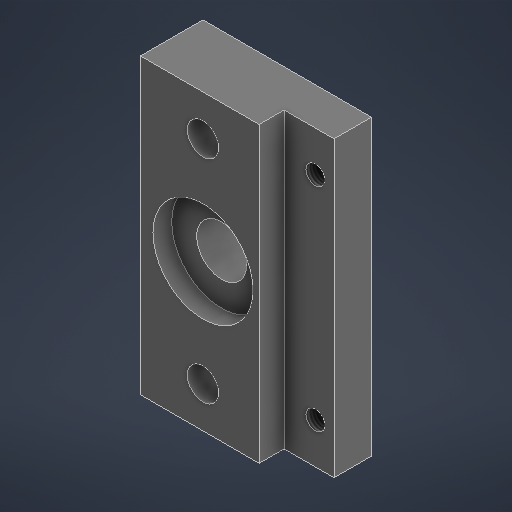
# Autodesk Inventor part: Szorítólap
Saved by Autodesk Inventor 2025 (Build 290162010, 162A)
## iProperties
Created: 2025-02-13
Part Number: Szorítólap
Material: Generic
Document SubType Name: Modeling
Designer: petruska.milan
Density: 1 g/cm^3
Appearance: Gray
Author: petruska.milan
Autodesk Inventor part; units mm, degrees
ref_plane "YZ Plane" through (0, 0, 0) normal (1, 0, 0) x (0, 1, 0)
ref_plane "XZ Plane" through (0, 0, 0) normal (0, 1, 0) x (-1, 0, 0)
ref_plane "XY Plane" through (0, 0, 0) normal (0, 0, 1) x (1, 0, 0)
sketch "Sketch1" plane through (0, 0, 0) normal (0, 0, 1) x (1, 0, 0)
  line L0 (-13.5, -23.5) -> (13.5, -23.5)
  line L1 (13.5, -23.5) -> (13.5, 23.5)
  line L2 (13.5, 23.5) -> (-13.5, 23.5)
  line L3 (-13.5, 23.5) -> (-13.5, -23.5)
  line L4 (-13.5, -23.5) -> (13.5, 23.5) construction
  line L5 (13.5, -23.5) -> (-13.5, 23.5) construction
  point P0 (0, 0)
  dimension "d0" = 27
  dimension "d1" = 47
  constraints: 12 end point, 2 midpoint, 2 parallel, 1 horizontal, 1 perpendicular
  measures "d0" distance of L2.end L1.end
  measures "d1" distance of L1.end L0.end
extrude "Extrusion1" add sketch "Sketch1" along normal blind 10
sketch "Sketch2" plane through (0, 0, 10) normal (0, 0, 1) x (1, 0, 0)
  line L0 (13.5, -23.5) -> (13.5, 23.5) projected
  line L1 (13.5, 23.5) -> (10.5, 23.5)
  line L2 (13.5, 23.5) -> (-13.5, 23.5) projected
  line L3 (10.5, 23.5) -> (10.5, 17)
  line L4 (10.5, 17) -> (10.5, -17)
  circle A0 centre (10.5, -17) radius 1.5
  circle A1 centre (10.5, 17) radius 1.5
  line L5 (13.5, 23.5) -> (10.5, 23.5)
  line L6 (13.5, 23.5) -> (-3.5, 23.5)
  line L7 (-3.5, 23.5) -> (-3.5, 17)
  circle A2 centre (-3.5, 17) radius 2.5
  line L8 (-3.5, 23.5) -> (-3.5, 0)
  circle A3 centre (-3.5, 0) radius 4
  line L9 (-3.5, 0) -> (-3.5, -15.5)
  line L10 (-3.5, -15.5) -> (-3.5, -17)
  circle A4 centre (-3.5, -17) radius 2.5
  point P0 (0, 0)
  dimension "d4" = 3
  dimension "d5" = 6.5
  dimension "d6" = 34
  dimension "d7" = 3
  dimension "d8" = 3
  dimension "d9" = 17
  dimension "d10" = 6.5
  dimension "d11" = 5
  dimension "d12" = 8
  dimension "d13" = 5
  constraints: 18 end point, 5 centre point, 5 coincident, 3 point on line, 3 vertical, 2 perpendicular, 1 collinear
  measures "d4" distance of L0.end L1.end
  measures "d5" distance of L1.end L3.end
  measures "d6" distance of L3.end L4.end
  measures "d7" diameter of A0
  measures "d8" diameter of A1
  measures "d9" distance of L0.end L6.end
  measures "d10" distance of L6.end L7.end
  measures "d11" diameter of A2
  measures "d12" diameter of A3
  measures "d13" diameter of A4
extrude "Extrusion2" cut sketch "Sketch2" against normal through all
sketch "Sketch3" plane through (0, 0, 10) normal (0, 0, 1) x (1, 0, 0)
  circle A0 centre (-3.5, 0) radius 4 projected
  circle A1 centre (-3.5, 0) radius 8
  point P0 (0, 0)
  dimension "d16" = 16
  constraints: 1 centre point, 1 coincident
  measures "d16" diameter of A1
extrude "Extrusion3" cut sketch "Sketch3" against normal blind 3
sketch "Sketch4" plane through (0, 0, 10) normal (0, 0, 1) x (1, 0, 0)
  line L0 (13.5, -23.5) -> (13.5, 23.5) projected
  line L1 (-13.5, -23.5) -> (13.5, -23.5) projected
  line L2 (13.5, 23.5) -> (5.5, 23.5)
  line L3 (5.5, 23.5) -> (5.5, -23.5)
  line L4 (5.5, -23.5) -> (13.5, -23.5)
  line L5 (13.5, -23.5) -> (13.5, 23.5)
  point P0 (0, 0)
  dimension "d19" = 8
  constraints: 8 end point, 2 parallel, 1 horizontal, 1 perpendicular, 1 point on line
  measures "d19" distance of L4.end L3.end
extrude "Extrusion4" cut sketch "Sketch4" against normal blind 4
thread "Thread1" size "M3x0.5" class "6H" standard "ANSI Metric M Profile" length 50
thread "Thread2" size "M3x0.5" class "6H" standard "ANSI Metric M Profile" length 50
body "Solid1"
